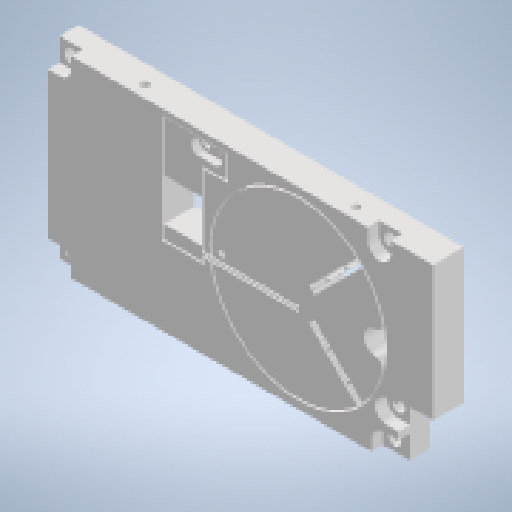
# Autodesk Inventor part: RoueV3PartC
Saved by Autodesk Inventor 2023 (Build 270158000, 158)
## iProperties
Created: 2023-04-29
Part Number: RoueV3PartC
Material: Generic
Document SubType Name: Modeling
Designer: Nathann
Density: 1 g/cm^3
Appearance: Default
Author: Nathann
Autodesk Inventor part; units mm, degrees
ref_plane "YZ Plane" through (0, 0, 0) normal (1, 0, 0) x (0, 1, 0)
ref_plane "XZ Plane" through (0, 0, 0) normal (0, 1, 0) x (-1, 0, 0)
ref_plane "XY Plane" through (0, 0, 0) normal (0, 0, 1) x (1, 0, 0)
sketch "Sketch1" plane through (0, 0, 0) normal (0, 0, 1) x (1, 0, 0)
  line L0 (50, -25) -> (50, 25) projected
  line L1 (50, 25) -> (-50, 25) projected
  line L2 (-50, 25) -> (-50, -25) projected
  line L3 (-50, -25) -> (50, -25) projected
  circle A0 centre (35, -20) radius 1.75 projected
  circle A1 centre (35, 20) radius 1.75 projected
  circle A2 centre (-45, -20) radius 1.75 projected
  circle A3 centre (-45, 20) radius 1.75 projected
  point P0 (0, 0)
extrude "Extrusion1" add sketch "Sketch1" along normal blind 8 contours L3 L2 L1 L0 | A0 | A1 | A2 | A3
sketch "Sketch2" plane through (0, 0, 8) normal (0, 0, 1) x (1, 0, 0)
  line L0 (-50, -25) -> (50, -25) projected
  line L1 (50, -25) -> (41, -25)
  line L2 (41, -25) -> (41, -10)
  line L3 (41, -10) -> (50, -10)
  line L4 (50, -10) -> (50, -25)
  point P0 (0, 0)
  point P1 (50, -17.5)
  dimension "d2" = 9
  dimension "d3" = 15
  constraints: 8 end point, 2 parallel, 1 horizontal, 1 midpoint, 1 perpendicular
  measures "d2" distance from line of point (50, -17.5) L2
  measures "d3" distance between parallel lines of L0 L3
extrude "Extrusion2" cut sketch "Sketch2" against normal blind 9
sketch "Sketch3" plane through (0, 0, 8) normal (0, 0, 1) x (1, 0, 0)
  circle A0 centre (35, 0) radius 3
  circle A1 centre (-5, 0) radius 0.8
  line L0 (50, -10) -> (50, 25) projected
  circle A2 centre (15, 0) radius 22.5
  line L1 (15, 0) -> (-7.3345, 22.3345)
  line L2 (15, 0) -> (5.2633, 0)
  line L3 (15, 0) -> (-4.6856, -19.6856)
  circle A3 centre (15, 0) radius 5
  circle A4 centre (15, 0) radius 23
  line L4 (10.8288, 2.757) -> (-1.6013, 15.1871)
  line L5 (12.243, 4.1712) -> (-0.1871, 16.6013)
  line L6 (10.8288, -2.757) -> (-1.6013, -15.1871)
  line L7 (-0.1871, -16.6013) -> (12.243, -4.1712)
  line L8 (11.4293, -3.5) -> (-1.2988, -16.2281)
  line L9 (-1.2281, -16.2988) -> (11.5, -3.5707)
  line L10 (11.4293, 3.5) -> (-1.2988, 16.2281)
  line L11 (-1.2281, 16.2988) -> (11.5, 3.5707)
  line L12 (15, -22.5) -> (15, -7.0707)
  line L13 (15, 0) -> (37.3345, 22.3345)
  line L14 (15, 0) -> (34.6856, -19.6856)
  line L15 (19.1712, 2.757) -> (31.6013, 15.1871)
  line L16 (17.757, 4.1712) -> (30.1871, 16.6013)
  line L17 (19.1712, -2.757) -> (31.6013, -15.1871)
  line L18 (30.1871, -16.6013) -> (17.757, -4.1712)
  line L19 (18.5707, -3.5) -> (31.2988, -16.2281)
  line L20 (31.2281, -16.2988) -> (18.5, -3.5707)
  line L21 (18.5707, 3.5) -> (31.2988, 16.2281)
  line L22 (31.2281, 16.2988) -> (18.5, 3.5707)
  circle A5 centre (22.7067, -6.2925) radius 0.95
  circle A6 centre (24.121, -7.7067) radius 0.95
  circle A7 centre (27.6565, -11.2423) radius 0.95
  circle A8 centre (29.0707, -12.6565) radius 0.95
  circle A9 centre (26.2423, 12.6565) radius 0.95
  circle A10 centre (22.7067, 9.121) radius 0.95
  circle A11 centre (21.2925, 7.7067) radius 0.95
  circle A12 centre (27.6565, 14.0707) radius 0.95
  point P0 (0, 0)
  point P1 (37.4312, 1.7576)
  point P2 (37.4312, -1.7576)
  point P3 (31.2281, -16.2988)
  point P4 (18.5, -3.5707)
  point P5 (18.5, 3.5707)
  point P6 (31.2281, 16.2988)
  point P7 (31.2988, 16.2281)
  point P8 (18.5707, 3.5)
  point P9 (18.5707, -3.5)
  point P10 (31.2988, -16.2281)
  point P11 (22.035, -6.9643)
  point P12 (23.3785, -6.9643)
  point P13 (23.4492, -7.035)
  point P14 (23.4492, -8.3785)
  point P15 (26.9847, -11.914)
  point P16 (28.3282, -11.914)
  point P17 (28.399, -11.9847)
  point P18 (28.399, -13.3282)
  point P19 (23.3785, 8.4492)
  point P20 (26.914, 11.9847)
  point P21 (26.914, 13.3282)
  point P22 (22.035, 8.4492)
  point P23 (21.9643, 7.035)
  point P24 (21.9643, 8.3785)
  point P25 (28.3282, 13.399)
  point P26 (26.9847, 13.399)
  dimension "d14" = 10
  dimension "d6" = 15
  dimension "d7" = 40
  dimension "d8" = 1.6
  dimension "d9" = 6
  dimension "d10" = 45
  dimension "d11" = 20
  dimension "d12" = 45
  dimension "d13" = 45
  dimension "d15" = 46
  dimension "d16" = 1
  dimension "d17" = 1
  dimension "d18" = 1
  dimension "d19" = 1
  dimension "d20" = 0.05
  dimension "d21" = 0.1
  dimension "d22" = 0.1
  dimension "d23" = 0.05
  dimension "d116" = 5
  dimension "d117" = 2
  dimension "d118" = 5
  dimension "d119" = 2
  dimension "d120" = 5
  dimension "d121" = 2
  dimension "d122" = 5
  dimension "d123" = 2
  constraints: 44 end point, 18 symmetric about line, 12 centre point, 9 point on circle, 8 point on line, 8 tangent, 5 parallel, 2 coincident, 1 horizontal, 1 vertical, 10 other
  measures "d6" distance from line of L0 A0.centre
  measures "d7" distance of A0.centre A1.centre
  measures "d8" diameter of A1
  measures "d9" diameter of A0
  measures "d10" diameter of A2
  measures "d11" distance of L1.start A1.centre
  measures "d12" angle of L2 L3
  measures "d13" angle of L1 L2
  measures "d15" diameter of A4
  measures "d16" distance between parallel lines of L1 L4
  measures "d17" distance between parallel lines of L5 L1
  measures "d18" distance between parallel lines of L3 L6
  measures "d19" distance between parallel lines of L7 L3
  measures "d20" distance between parallel lines of L3 L8
  measures "d21" distance between parallel lines of L9 L8
  measures "d22" distance between parallel lines of L11 L10
  measures "d23" distance between parallel lines of L1 L10
  measures "d116" distance of A5.centre L17.start
  measures "d117" distance of A5.centre A6.centre
  measures "d118" distance of A6.centre A7.centre
  measures "d119" distance of A7.centre A8.centre
  measures "d120" distance of L16.start A11.centre
  measures "d121" distance of A10.centre A11.centre
  measures "d122" distance of A9.centre A10.centre
  measures "d123" distance of A9.centre A12.centre
extrude "Extrusion3" cut sketch "Sketch3" against normal blind 8 contours A0 A2 | A4 L19 A2 A0 | A0 A2 L21 A4 | A2 A0 | L15 A3 L21 A2 | A2 L19 A8 L17 | A8 L17 | L22 A2 L11 A4 | A4 L9 A2 L20 | L11 A2 L1 A4 | L22 A12 L16 A2 | A4 L3 A2 L9 | A2 L18 A3 L20 | L19 A6 L17 A7 | A7 L17 | L17 A5 L19 A3 | L1 A2 L10 A4 | A12 L16 | A3 L16 A11 L22 | A4 L8 A2 L3 | A6 L17 | L17 A5 | L10 A2 L8 A4 | L22 A10 L16 A9 | A9 L16 | A11 L16 | A10 L16 | A1 picked at (28.9107, -12.9996) picked at (27.825, -11.5104) picked at (27.5519, 13.7718) picked at (23.7532, -7.9749) picked at (22.4078, -6.1879) picked at (26.8341, 12.3096) picked at (21.3125, 7.3478) picked at (23.0628, 8.7211)
fillet "Fillet1" radius 2 2 edges at (37.4312, 1.7576, 4) (37.4312, -1.7576, 4)
sketch "Sketch4" plane through (0, 0, 8) normal (0, 0, 1) x (1, 0, 0)
  arc A0 (36.8209, 5.4863) -> (31.6013, 15.1871) centre (15, 0) ccw projected
  line L0 (50, 25) -> (-50, 25) projected
  line L1 (15, -2.25) -> (-13.8792, -2.25)
  line L2 (-13.8792, -2.25) -> (-13.8792, -2.65)
  line L3 (-13.8792, -2.65) -> (15, -2.65)
  line L4 (15, -2.65) -> (15, -2.25)
  line L5 (-10, -4.15) -> (-20, -4.15)
  line L6 (-20, -4.15) -> (-20, -0.75)
  line L7 (-20, -0.75) -> (-10, -0.75)
  line L8 (-10, -0.75) -> (-10, -4.15)
  line L9 (-20, -0.75) -> (-19.9, -0.75)
  line L10 (-19.9, -0.75) -> (-19.9, 17.25)
  line L11 (-19.9, 17.25) -> (-20, 17.25)
  line L12 (-20, 17.25) -> (-20, -0.75)
  line L13 (-20, 17.25) -> (-4, 17.25)
  line L14 (-4, 17.25) -> (-4, 25)
  line L15 (-4, 25) -> (-20, 25)
  line L16 (-20, 25) -> (-20, 17.25)
  line L17 (15, -2.65) -> (-10, -2.65)
  line L18 (-10, -2.65) -> (-10, -3.15)
  line L19 (-10, -3.15) -> (15, -3.15)
  line L20 (15, -3.15) -> (15, -2.65)
  line L21 (15, -2.25) -> (-10, -2.25)
  line L22 (-10, -2.25) -> (-10, -1.75)
  line L23 (-10, -1.75) -> (15, -1.75)
  line L24 (15, -1.75) -> (15, -2.25)
  circle A1 centre (-5, 0) radius 0.8 projected
  line L25 (-10, -0.75) -> (-10.1, -0.75)
  line L26 (-10.1, -0.75) -> (-10.1, 17.25)
  line L27 (-10.1, 17.25) -> (-10, 17.25)
  line L28 (-10, 17.25) -> (-10, -0.75)
  line L29 (-10, -1.75) -> (-9.5, -1.75)
  line L30 (-9.5, -1.75) -> (-9.5, 17.25)
  line L31 (-9.5, 17.25) -> (-10, 17.25)
  line L32 (-10, 17.25) -> (-10, -1.75)
  line L33 (-20, 17.25) -> (-20.5, 17.25)
  line L34 (-20.5, 17.25) -> (-20.5, -4.15)
  line L35 (-20.5, -4.15) -> (-20, -4.15)
  line L36 (-20, -4.15) -> (-20, 17.25)
  line L37 (-20.5, -4.15) -> (-9.5, -4.15)
  line L38 (-9.5, -4.15) -> (-9.5, -4.65)
  line L39 (-9.5, -4.65) -> (-20.5, -4.65)
  line L40 (-20.5, -4.65) -> (-20.5, -4.15)
  line L41 (-10, -3.15) -> (-9.5, -3.15)
  line L42 (-9.5, -3.15) -> (-9.5, -4.15)
  line L43 (-9.5, -4.15) -> (-10, -4.15)
  line L44 (-10, -4.15) -> (-10, -3.15)
  line L45 (-9.5, 17.25) -> (-3.5, 17.25)
  line L46 (-3.5, 17.25) -> (-3.5, 16.75)
  line L47 (-3.5, 16.75) -> (-9.5, 16.75)
  line L48 (-9.5, 16.75) -> (-9.5, 17.25)
  line L49 (-3.5, 17.25) -> (-4, 17.25)
  line L50 (-4, 17.25) -> (-4, 25)
  line L51 (-4, 25) -> (-3.5, 25)
  line L52 (-3.5, 25) -> (-3.5, 17.25)
  line L53 (-20, 25) -> (-20.5, 25)
  line L54 (-20.5, 25) -> (-20.5, 19.7674)
  line L55 (-20.5, 19.7674) -> (-20, 19.7674)
  line L56 (-20, 19.7674) -> (-20, 25)
  line L57 (-20, 19.7674) -> (-20.5, 19.7674)
  line L58 (-20.5, 19.7674) -> (-20.5, 17.25)
  line L59 (-20.5, 17.25) -> (-20, 17.25)
  line L60 (-20, 17.25) -> (-20, 19.7674)
  line L61 (-3.5, 23.5) -> (-20.5, 23.5)
  line L62 (-20.5, 23.5) -> (-20.5, 23.4)
  line L63 (-20.5, 23.4) -> (-3.5, 23.4)
  line L64 (-3.5, 23.4) -> (-3.5, 23.5)
  line L65 (-19.9, 17.25) -> (-10.1, 17.25)
  line L66 (-10.1, 17.25) -> (-10.1, 10.25)
  line L67 (-10.1, 10.25) -> (-19.9, 10.25)
  line L68 (-19.9, 10.25) -> (-19.9, 17.25)
  circle A2 centre (-11.1, 3.7) radius 1
  circle A3 centre (-11.1, 5.8) radius 1
  circle A4 centre (-18.9, 5.8) radius 1
  circle A5 centre (-18.9, 3.7) radius 1
  line L69 (-11.1, 2.7) -> (-18.9, 2.7)
  line L70 (-11.1, 6.8) -> (-18.9, 6.8)
  line L71 (-11.1, 2.7) -> (-11.1, 4.7)
  line L72 (-11.1, 4.8) -> (-11.1, 6.8)
  line L73 (-18.9, 6.8) -> (-18.9, 4.8)
  line L74 (-18.9, 4.7) -> (-18.9, 2.7)
  line L75 (-12.1, 3.7) -> (-12.1, 2.7)
  line L76 (-17.9, 3.7) -> (-17.9, 2.7)
  line L77 (-12.1, 5.8) -> (-12.1, 6.8)
  line L78 (-17.9, 5.8) -> (-17.9, 6.8)
  point P0 (-0.1871, -16.6013)
  point P1 (36.8209, -5.4863)
  point P2 (-10, -2.9)
  point P3 (-10.1, -0.75)
  point P4 (-19.9, -0.75)
  point P5 (-10, -2.65)
  point P6 (-20, 23.4)
  point P7 (-4, 23.4)
  point P8 (-4, 23.5)
  point P9 (-23.0406, 20.2674)
  point P10 (-4, 17.25)
  point P11 (-4, 17.25)
  point P12 (-3.5, 23.4)
  point P13 (-20, 23.5)
  point P14 (-20, 25)
  point P15 (-12, 17.25)
  point P16 (-10.1, 5.8)
  point P17 (-19.9, 5.8)
  point P18 (-19.9, 3.7)
  point P19 (-10.1, 3.7)
  dimension "d33" = 2.65
  dimension "d34" = 0.4
  dimension "d35" = 0.5
  dimension "d36" = 0.5
  dimension "d37" = 20
  dimension "d38" = 1.75
  dimension "d39" = 1.6
  dimension "d40" = 25
  dimension "d41" = 0
  dimension "d42" = 0.5
  dimension "d43" = 0.5
  dimension "d44" = 0.5
  dimension "d45" = 0.5
  dimension "d47" = 1.5
  dimension "d48" = 1.5
  dimension "d49" = 0.1
  dimension "d50" = 0.1
  dimension "d51" = 0.5
  dimension "d52" = 0.5
  dimension "d53" = 0.5
  dimension "d54" = 18
  dimension "d56" = 0
  dimension "d57" = 1.5
  dimension "d58" = 0.1
  dimension "d63" = 16
  dimension "d108" = 10
  dimension "d115" = 7
  dimension "d124" = 11
  dimension "d125" = 1
  dimension "d126" = 1
  dimension "d127" = 2.1
  dimension "d128" = 4.45
  dimension "d129" = 2
  dimension "d130" = 2
  dimension "d131" = 4.45
  dimension "d132" = 2.1
  constraints: 156 end point, 36 equal length, 22 point on line, 19 perpendicular, 17 horizontal, 12 point on circle, 7 tangent, 4 centre point, 2 midpoint, 1 vertical
  measures "d33" distance from line of A0.centre L3
  measures "d34" distance between parallel lines of L3 L1
  measures "d35" distance between parallel lines of L3 L19
  measures "d36" distance between parallel lines of L1 L23
  measures "d37" distance of A0.centre A1.centre
  measures "d38" distance from line of L23 A1.centre
  measures "d39" diameter of A1
  measures "d40" distance of L18.end L19.end
  measures "d41" horizontal distance of A0.centre L19.end
  measures "d42" distance between parallel lines of L32 L30
  measures "d43" distance between parallel lines of L6 L34
  measures "d44" distance between parallel lines of L43 L39
  measures "d45" distance between parallel lines of L8 L42
  measures "d47" distance between parallel lines of L5 L3
  measures "d48" distance between parallel lines of L7 L1
  measures "d49" distance between parallel lines of L26 L28
  measures "d50" distance between parallel lines of L36 L10
  measures "d51" distance between parallel lines of L47 L13
  measures "d52" distance between parallel lines of L14 L52
  measures "d53" distance between parallel lines of L54 L16
  measures "d54" distance of L11.end L9.start
  measures "d56" distance between parallel lines of L16 L36
  measures "d57" distance between parallel lines of L0 L61
  measures "d58" distance between parallel lines of L61 L63
  measures "d63" distance between parallel lines of L16 L14
  measures "d108" distance between parallel lines of L6 L8
  measures "d115" distance from line of point (-12, 17.25) L67
  measures "d124" distance between parallel lines of L67 L7
  measures "d125" distance from line of L26 A3.centre
  measures "d126" distance from line of L26 A2.centre
  measures "d127" distance of A3.centre A2.centre
  measures "d128" distance from line of L67 A3.centre
  measures "d129" diameter of A5
  measures "d130" diameter of A4
  measures "d131" distance from line of L67 A4.centre
  measures "d132" distance of A4.centre A5.centre
extrude "Extrusion4" cut sketch "Sketch4" against normal blind 8 contours L52 L61 L14 L0 | L52 L63 L14 L61 | L14 L63 L16 L61 | L52 L45 L14 L63 | L16 L63 L54 L61 | L46 L47 L30 L13 L45 | L16 L55 L54 L63 | L16 L33 L58 L55 | L30 L23 L8 L28 L13 | L12 L6 L35 L34 L33 | L23 L24 L1 L8 | L35 L5 L37 L38 L39 L40 | L67 L26 A3 L70 A4 L10 | L10 A5 L69 A2 L26 L7 | A4 L73 | L8 L19 L42 L37 | A5 L74 | A3 L72 | A2 L71 | L3 L20 L19 L8 | L70 L78 A4 | A4 L73 | A5 L74 | A5 L76 L69 | L72 A3 | A3 L77 L70 | L71 A2 | L69 L75 A2
sketch "Sketch5" plane through (0, 0, 8) normal (0, 0, 1) x (1, 0, 0)
  line L0 (-7.8468, -2.65) -> (-10, -2.65) projected
  line L1 (15, -2.25) -> (-7.3872, -2.25) projected
  line L2 (-8.0927, -2.65) -> (-6.7574, -2.65)
  line L3 (-6.7574, -2.65) -> (-6.7574, -2.25)
  line L4 (-6.7574, -2.25) -> (-8.0927, -2.25)
  line L5 (-8.0927, -2.25) -> (-8.0927, -2.65)
  line L6 (-4, 25) -> (-4, 23.5) projected
  line L7 (-3.5, 16.75) -> (-3.5, 25) projected
  line L8 (-4, 23.5) -> (-3.5, 23.5)
  line L9 (-3.5, 23.5) -> (-3.5, 25)
  line L10 (-3.5, 25) -> (-4, 25)
  line L11 (-4, 25) -> (-4, 23.5)
  point P0 (0, 0)
  point P1 (-3.5, 23.5)
  constraints: 16 end point, 4 parallel, 2 horizontal, 2 perpendicular, 2 point on line
extrude "Extrusion5" add sketch "Sketch5" against normal blind 8
sketch "Sketch7" plane through (0, 0, 8) normal (0, 0, 1) x (1, 0, 0)
  circle A0 centre (-6.7879, 21) radius 0.8 projected
  circle A1 centre (-10.7879, 21) radius 0.8 projected
  circle A2 centre (-6.7879, 21) radius 1.2
  circle A3 centre (-10.7879, 21) radius 1.2
  point P0 (0, 0)
  dimension "d64" = 2.4
  dimension "d65" = 2.4
  constraints: 2 centre point, 2 coincident
  measures "d64" diameter of A2
  measures "d65" diameter of A3
extrude "Extrusion6" cut sketch "Sketch7" against normal blind 8 contours A0 | A1 | A2 | A3
sketch "Sketch8" plane through (0, 0, 8) normal (0, 0, 1) x (1, 0, 0)
  circle A0 centre (36, 22) radius 1.7
  line L0 (50, 25) -> (-50, 25) projected
  line L1 (50, -10) -> (50, 25) projected
  circle A1 centre (-47, 22) radius 1.7
  line L2 (-50, 25) -> (-50, -25) projected
  circle A2 centre (-47, -22) radius 1.7
  line L3 (-50, -25) -> (41, -25) projected
  circle A3 centre (37, -22) radius 1.7
  line L4 (41, -25) -> (41, -10) projected
  circle A4 centre (38, -14) radius 1.7
  point P0 (0, 0)
  dimension "d68" = 3
  dimension "d69" = 14
  dimension "d70" = 3
  dimension "d72" = 3
  dimension "d73" = 3.4
  dimension "d74" = 3.4
  dimension "d75" = 3.4
  dimension "d76" = 3
  dimension "d77" = 3
  dimension "d78" = 3
  dimension "d79" = 4
  dimension "d80" = 3.4
  dimension "d81" = 3
  dimension "d82" = 3.4
  dimension "d83" = 11
  constraints: 5 centre point
  measures "d68" distance from line of L0 A0.centre
  measures "d69" distance from line of L1 A0.centre
  measures "d70" distance from line of A1.centre L0
  measures "d72" distance from line of A1.centre L2
  measures "d73" diameter of A1
  measures "d74" diameter of A0
  measures "d75" diameter of A2
  measures "d76" distance from line of L2 A2.centre
  measures "d77" distance from line of A2.centre L3
  measures "d78" distance from line of A3.centre L3
  measures "d79" distance from line of L4 A3.centre
  measures "d80" diameter of A3
  measures "d81" distance from line of L4 A4.centre
  measures "d82" diameter of A4
  measures "d83" distance from line of L3 A4.centre
extrude "Extrusion7" cut sketch "Sketch8" against normal blind 8
sketch "Sketch10" plane through (0, 0, 8) normal (0, 0, 1) x (1, 0, 0)
  circle A0 centre (37, -22) radius 1.7 projected
  circle A1 centre (37, -22) radius 3
  circle A2 centre (38, -14) radius 1.7 projected
  circle A3 centre (38, -14) radius 3
  circle A4 centre (36, 22) radius 1.7 projected
  circle A5 centre (36, 22) radius 3
  circle A6 centre (-47, -22) radius 1.7 projected
  circle A7 centre (-47, -22) radius 3
  circle A8 centre (-47, 22) radius 1.7 projected
  circle A9 centre (-47, 22) radius 3
  line L0 (50, 25) -> (-50, 25) projected
  line L1 (-50, 25) -> (-47, 25)
  line L2 (-47, 25) -> (-47, 22)
  line L3 (-47, 22) -> (-50, 22)
  line L4 (-50, 22) -> (-50, 25)
  line L5 (-50, -25) -> (41, -25) projected
  line L6 (-47, -22) -> (-50, -22)
  line L7 (-50, -22) -> (-50, -25)
  line L8 (-50, -25) -> (-47, -25)
  line L9 (-47, -25) -> (-47, -22)
  line L10 (37, -22) -> (41, -22)
  line L11 (41, -22) -> (41, -25)
  line L12 (41, -25) -> (37, -25)
  line L13 (37, -25) -> (37, -22)
  line L14 (41, -10) -> (41, -25) projected
  line L15 (38, -17) -> (41, -17)
  line L16 (41, -17) -> (41, -11)
  line L17 (41, -11) -> (38, -11)
  line L18 (38, -11) -> (38, -17)
  line L19 (39, 22) -> (33, 22)
  line L20 (33, 22) -> (33, 25)
  line L21 (33, 25) -> (39, 25)
  line L22 (39, 25) -> (39, 22)
  line L23 (37, -22) -> (34, -22)
  line L24 (34, -22) -> (34, -25)
  line L25 (34, -25) -> (37, -25)
  line L26 (37, -25) -> (37, -22)
  line L27 (-50, -25) -> (41, -25) projected
  line L28 (-47, -22) -> (-44, -22)
  line L29 (-44, -22) -> (-44, -25)
  line L30 (-44, -25) -> (-47, -25)
  line L31 (-47, -25) -> (-47, -22)
  line L32 (-47, -22) -> (-50, -22)
  line L33 (-50, -22) -> (-50, -19)
  line L34 (-50, -19) -> (-47, -19)
  line L35 (-47, -19) -> (-47, -22)
  circle A10 centre (-47, 22) radius 1.7 projected
  line L36 (-50, 25) -> (-50, -25) projected
  line L37 (-47, 22) -> (-50, 22)
  line L38 (-50, 22) -> (-50, 19)
  line L39 (-50, 19) -> (-47, 19)
  line L40 (-47, 19) -> (-47, 22)
  line L41 (-47, 22) -> (-44, 22)
  line L42 (-44, 22) -> (-44, 25.1289)
  line L43 (-44, 25.1289) -> (-47, 25.1289)
  line L44 (-47, 25.1289) -> (-47, 22)
  line L45 (41, -22) -> (37, -22)
  line L46 (37, -22) -> (37, -19)
  line L47 (37, -19) -> (41, -19)
  line L48 (41, -19) -> (41, -22)
  point P0 (0, 0)
  point P1 (-47, -25)
  point P2 (-47, 25)
  point P3 (36, 25)
  point P4 (38, -12.3)
  point P5 (38, -15.7)
  point P6 (41, -14)
  point P7 (33, -22)
  point P8 (37, -25)
  point P9 (40, -22)
  point P10 (-44, 25)
  point P11 (37, -25)
  dimension "d87" = 6
  dimension "d88" = 6
  dimension "d86" = 6
  dimension "d89" = 6
  dimension "d90" = 6
  constraints: 88 end point, 22 parallel, 11 horizontal, 11 perpendicular, 6 point on line, 5 coincident, 3 centre point, 2 point on circle, 6 other
  measures "d86" diameter of A1
  measures "d89" diameter of A7
  measures "d90" diameter of A9
extrude "Extrusion8" cut sketch "Sketch10" against normal blind 3 contours L10 A1 L13 A0 | A0 L46 A1 L10 | A0 L23 A1 L46 | L13 A1 L23 A0 | L10 L11 L5 A1 | A1 L47 L14 L10 | L5 L24 A1 | A2 L18 | A2 L18 A3 | A2 L18 A3 | L17 L14 A3 | A3 L14 L15 | L19 A4 | L19 A5 A4 | A4 L19 A5 | A4 L19 | A5 L0 L22 | L20 L0 A5 | L28 L35 A6 | L28 A7 L9 A6 | A6 L9 L28 | A6 L35 A7 L28 | L35 L6 A6 | A6 L6 A7 L35 | L9 A7 L6 A6 | A6 L6 L9 | L29 L5 A7 | A7 L33 L34 | L5 L7 A7 | L41 L2 A8 | L41 A9 L40 A8 | A8 L40 L41 | A8 L2 A9 L41 | L2 L3 A8 | A8 L3 A9 L2 | L40 A9 L3 A8 | A8 L3 L40 | A9 L0 L42 | A9 L4 L0 | L39 L36 A9 picked at (38.3533, -13.557)
sketch "Sketch11" plane through (0, 0, 8) normal (0, 0, 1) x (1, 0, 0)
  circle A0 centre (-6.7879, 21) radius 1.2 projected
  circle A1 centre (-6.7879, 21) radius 2
  circle A2 centre (-10.7879, 21) radius 1.2 projected
  circle A3 centre (-10.7879, 21) radius 2
  line L0 (-6.7879, 19) -> (-10.7879, 19)
  line L1 (-6.7879, 23) -> (-10.7879, 23)
  point P0 (0, 0)
  point P1 (-8.7879, 21)
  dimension "d93" = 4
  dimension "d94" = 4
  constraints: 4 end point, 4 point on circle, 2 centre point, 2 coincident, 2 tangent
  measures "d93" diameter of A1
  measures "d94" diameter of A3
extrude "Extrusion9" cut sketch "Sketch11" against normal blind 2 contours A0 | A1 | A1 A3 L1 | L0 A3 A1 | A3
sketch "Sketch12" plane through (-50, -25, 0) normal (0, -1, 0) x (1, 0, 0)
  circle A0 centre (22, 5) radius 1.375
  circle A1 centre (77, 5) radius 1.375
  circle A2 centre (77, 5) radius 1.025
  circle A3 centre (22, 5) radius 1.025
  circle A4 centre (26.6377, -9) radius 1.375 projected
  circle A5 centre (81.6377, -9) radius 1.375 projected
  circle A6 centre (26.6377, -9) radius 1.025
  circle A7 centre (81.6377, -9) radius 1.025
  line L0 (100, 8) -> (100, 0) projected
  point P0 (50, 0)
  dimension "d99" = 2.05
  dimension "d100" = 2.75
  dimension "d101" = 2.05
  dimension "d102" = 2.05
  dimension "d103" = 2.05
  dimension "d113" = 23
  dimension "d114" = 55
  constraints: 6 centre point, 4 coincident
  measures "d99" diameter of A3
  measures "d100" diameter of A0
  measures "d101" diameter of A2
  measures "d102" diameter of A6
  measures "d103" diameter of A7
  measures "d113" distance from line of A1.centre L0
  measures "d114" distance of A0.centre A1.centre
extrude "Extrusion10" cut sketch "Sketch12" against normal blind 7 contours A0 | A1 | A2 | A3
sketch "Sketch13" plane through (-50, 25, 0) normal (0, 1, 0) x (1, 0, 0)
  circle A0 centre (22, -5) radius 1.025
  circle A1 centre (77, -5) radius 1.375
  circle A2 centre (81.6377, 9) radius 1.375 projected
  circle A3 centre (26.6377, 9) radius 1.375 projected
  circle A4 centre (77, -5) radius 1.025
  circle A5 centre (26.6377, -5) radius 1.025
  line L0 (100, 0) -> (100, -8) projected
  point P0 (50, 0)
  dimension "d104" = 2.05
  dimension "d105" = 2.05
  dimension "d109" = 23
  dimension "d110" = 55
  dimension "d111" = 55
  dimension "d112" = 2.05
  constraints: 4 centre point
  measures "d104" diameter of A5
  measures "d105" diameter of A4
  measures "d109" distance from line of L0 A1.centre
  measures "d110" distance of A0.centre A4.centre
  measures "d111" distance of A1.centre A0.centre
  measures "d112" diameter of A0
extrude "Extrusion11" cut sketch "Sketch13" against normal blind 7 contours A0 | A4
equation "\"d11\" = 0.5 * d7"
equation "\"d20\" = 0.5 * d21"
equation "\"d21\" = BladeThicknessRCC"
equation "\"d22\" = BladeThicknessRCC"
equation "\"d23\" = 0.5 * d22"
equation "\"d50\" = d49"
equation "\"bladeThicknessTablePushing\" = 0.1"
equation "\"bladeThicknessTable\" = 0.1"
equation "\"bladeThicknessForceConverter\" = 0.2"
equation "\"bladeThicknessWheelAnchor\" = 0.1"
equation "\"safetyPlay\" = 0.1"
equation "\"OffsetMotorSpring\" = -1"
equation "\"BladeThicknessRCC\" = 0.1"
equation "\"bladeThicknessZeroConverter\" = 0.1"
equation "\"rangeXProbeMin\" = -0.6"
equation "\"thicknessWheelPlate\" = 8"
equation "\"rangeXProbeMax\" = 0.6"
equation "\"BladeLengthRCC\" = 18"
equation "\"bladeLengthTable\" = 18"
equation "\"bladeLengthWheelAnchor\" = 7.5"
equation "\"RCCdeadCenter\" = 5"
equation "\"bladeLengthZeroConverter\" = 11.98"
equation "\"bladeLengthTablePushing\" = 12"
equation "\"bladeLengthForceConverter\" = 12.125"
equation "\"thicknessConverterPlate\" = 4"
body "Solid1"
